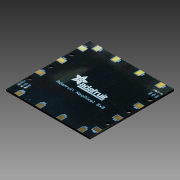
# Autodesk Inventor part: 8x8 board
Saved by Autodesk Inventor 2014 SP1 (Build 180222100, 222)
## iProperties
Created: 2014-04-19
Part Number: 8x8 board
Material: Acetal Resin, Black
Document SubType Name: Modeling
Designer: Ben
Density: 1.425 g/cm^3
Appearance: Smooth - Black
Author: Ben
Autodesk Inventor part; units mm, degrees
ref_plane "YZ Plane" through (0, 0, 0) normal (1, 0, 0) x (0, 1, 0)
ref_plane "XZ Plane" through (0, 0, 0) normal (0, 1, 0) x (-1, 0, 0)
ref_plane "XY Plane" through (0, 0, 0) normal (0, 0, 1) x (1, 0, 0)
sketch "Sketch1" plane through (0, 0, 0) normal (0, 0, 1) x (1, 0, 0)
  line L0 (0, 0) -> (71.17, 0)
  line L1 (71.17, 0) -> (71.17, 71.17)
  line L2 (71.17, 71.17) -> (0, 71.17)
  line L3 (0, 71.17) -> (0, 0)
  dimension "d0" = 71.17
  dimension "d1" = 71.17
  constraints: 8 end point, 2 parallel, 1 horizontal, 1 perpendicular
  measures "d0" distance of L2.end L1.end
  measures "d1" distance of L1.end L0.end
extrude "Extrusion1" add sketch "Sketch1" along normal blind 1.5
sketch "Sketch3" plane through (0, 0, 1.5) normal (0, 0, 1) x (1, 0, 0)
  line L0 (0, 71.17) -> (71.3183, 71.0211) construction
  line L1 (71.3183, 71.0211) -> (71.17, 0) construction
  line L2 (71.17, 0) -> (-0.1483, 0.1489) construction
  line L3 (-0.1483, 0.1489) -> (0, 71.17) construction
  constraints: 2 other
decal "Decal1"
sketch "Sketch4" plane through (0, 0, 0) normal (0, 0, -1) x (-1, 0, 0)
  line L0 (-71.17, 71.17) -> (0, 71.17) construction
  line L1 (0, 71.17) -> (0, 0) construction
  line L2 (0, 0) -> (-71.17, 0) construction
  line L3 (-71.17, 0) -> (-71.17, 71.17) construction
  constraints: 2 other
decal "Decal2"
sketch "Sketch5" plane through (0, 0, 1.5) normal (0, 0, 1) x (1, 0, 0)
  line L0 (0, 0) -> (71.17, 0) projected
  line L1 (71.17, 0) -> (71.17, 71.17) projected
  line L2 (71.17, 71.17) -> (0, 71.17) projected
  line L3 (71.17, 71.17) -> (0, 0)
  line L4 (0, 71.17) -> (71.17, 0)
  line L5 (35.585, 35.585) -> (35.585, 71.17)
  line L6 (71.17, 0) -> (71.17, 17.7925)
  line L7 (35.585, 35.585) -> (71.17, 35.585)
  line L8 (71.17, 71.17) -> (71.17, 53.3775)
  line L9 (35.585, 71.17) -> (68.585, 71.17)
  line L10 (68.585, 71.17) -> (68.585, 0)
  line L11 (71.17, 53.3775) -> (68.585, 53.3775)
  line L12 (71.17, 35.585) -> (68.585, 35.585)
  line L13 (71.17, 17.7925) -> (68.585, 17.7925)
  point P0 (2.585, 53.3775)
  point P1 (2.585, 35.585)
  point P2 (2.585, 17.7925)
  dimension "d25" = 17.7925
  dimension "d26" = 17.7925
  dimension "d27" = 33
  constraints: 22 end point, 6 point on line, 4 midpoint, 4 perpendicular, 3 coincident, 3 symmetric about line
  measures "d25" distance of L0.end L6.end
  measures "d26" distance of L1.end L8.end
  measures "d27" distance of L5.end L9.end
hole "Hole1" at (68.585, 53.3775, 1.5) at (68.585, 35.585, 1.5) at (68.585, 17.7925, 1.5) at (2.585, 53.3775, 1.5) at (2.585, 35.585, 1.5) at (2.585, 17.7925, 1.5) direction (0, 0, -1) diameter 3.2 end through all
body "Solid1"
